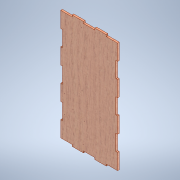
# Autodesk Inventor part: Costados pequeños
Saved by Autodesk Inventor 2020.3 (Build 243373000, 373)
## iProperties
Created: 2020-04-27
Part Number: Costados pequeños
Material: Madera (roble)
Document SubType Name: Modeling
Designer: miosh
Density: 0.76 g/cm^3
Appearance: Roble blanco - Natural brillo medio
Author: miosh
Autodesk Inventor part; units mm, degrees
ref_plane "YZ Plane" through (0, 0, 0) normal (1, 0, 0) x (0, 1, 0)
ref_plane "XZ Plane" through (0, 0, 0) normal (0, 1, 0) x (-1, 0, 0)
ref_plane "XY Plane" through (0, 0, 0) normal (0, 0, 1) x (1, 0, 0)
sketch "Boceto1" plane through (0, 0, 0) normal (0, 0, 1) x (1, 0, 0)
  line L0 (20, 0) -> (20, 3)
  line L1 (20, 3) -> (0, 3)
  line L2 (0, 3) -> (0, 30.71)
  line L3 (0, 30.71) -> (3, 30.71)
  line L4 (3, 30.71) -> (3, 58.43)
  line L5 (3, 58.43) -> (0, 58.43)
  line L6 (0, 58.43) -> (0, 86.14)
  line L7 (0, 86.14) -> (3, 86.14)
  line L8 (3, 86.14) -> (3, 113.86)
  line L9 (3, 113.86) -> (0, 113.86)
  line L10 (0, 113.86) -> (0, 141.57)
  line L11 (0, 141.57) -> (3, 141.57)
  line L12 (3, 141.57) -> (3, 169.29)
  line L13 (3, 169.29) -> (0, 169.29)
  line L14 (0, 169.29) -> (0, 197)
  line L15 (0, 197) -> (20, 197)
  line L16 (20, 197) -> (20, 200)
  line L17 (20, 200) -> (40, 200)
  line L18 (40, 200) -> (40, 197)
  line L19 (40, 197) -> (60, 197)
  line L20 (60, 197) -> (60, 200)
  line L21 (60, 200) -> (80, 200)
  line L22 (80, 200) -> (80, 197)
  line L23 (80, 197) -> (100, 197)
  line L24 (100, 197) -> (100, 169.29)
  line L25 (100, 169.29) -> (97, 169.29)
  line L26 (97, 169.29) -> (97, 141.57)
  line L27 (97, 141.57) -> (100, 141.57)
  line L28 (100, 141.57) -> (100, 113.86)
  line L29 (100, 113.86) -> (97, 113.86)
  line L30 (97, 113.86) -> (97, 86.14)
  line L31 (97, 86.14) -> (100, 86.14)
  line L32 (100, 86.14) -> (100, 58.43)
  line L33 (100, 58.43) -> (97, 58.43)
  line L34 (97, 58.43) -> (97, 30.71)
  line L35 (97, 30.71) -> (100, 30.71)
  line L36 (100, 30.71) -> (100, 3)
  line L37 (100, 3) -> (80, 3)
  line L38 (80, 3) -> (80, 0)
  line L39 (80, 0) -> (60, 0)
  line L40 (60, 0) -> (60, 3)
  line L41 (60, 3) -> (40, 3)
  line L42 (40, 3) -> (40, 0)
  line L43 (40, 0) -> (20, 0)
  point P0 (0, 0)
  dimension "d0" = 3
  dimension "d1" = 27.71
  dimension "d2" = 3
  dimension "d3" = 27.72
  dimension "d4" = 3
  dimension "d5" = 27.71
  dimension "d6" = 3
  dimension "d7" = 27.72
  dimension "d8" = 3
  dimension "d9" = 27.71
  dimension "d10" = 3
  dimension "d11" = 27.72
  dimension "d12" = 3
  dimension "d13" = 27.71
  dimension "d14" = 20
  dimension "d16" = 20
  dimension "d18" = 20
  dimension "d20" = 20
  dimension "d22" = 20
  dimension "d23" = 27.71
  dimension "d24" = 3
  dimension "d25" = 27.72
  dimension "d26" = 3
  dimension "d27" = 27.71
  dimension "d28" = 3
  dimension "d29" = 27.72
  dimension "d30" = 3
  dimension "d31" = 27.71
  dimension "d32" = 3
  dimension "d33" = 27.72
  dimension "d34" = 3
  dimension "d35" = 20
  dimension "d39" = 20
  dimension "d46" = 3
  dimension "d47" = 27.71
  dimension "d50" = 3
  constraints: 88 end point, 26 point on line, 13 perpendicular, 4 vertical, 1 horizontal
  measures "d0" distance of L0.start L0.end
  measures "d1" distance of L1.end L2.end
  measures "d2" distance of L2.end L3.end
  measures "d3" distance of L3.end L4.end
  measures "d4" distance of L4.end L5.end
  measures "d5" distance of L5.end L6.end
  measures "d6" distance of L6.end L7.end
  measures "d7" distance of L7.end L8.end
  measures "d8" distance of L8.end L9.end
  measures "d9" distance of L9.end L10.end
  measures "d10" distance of L10.end L11.end
  measures "d11" distance of L11.end L12.end
  measures "d12" distance of L12.end L13.end
  measures "d13" distance of L13.end L14.end
  measures "d14" distance of L14.end L15.end
  measures "d16" distance of L16.end L17.end
  measures "d18" distance of L18.end L19.end
  measures "d20" distance of L20.end L21.end
  measures "d22" distance of L22.end L23.end
  measures "d23" distance of L23.end L24.end
  measures "d24" distance of L24.end L25.end
  measures "d25" distance of L25.end L26.end
  measures "d26" distance of L26.end L27.end
  measures "d27" distance of L27.end L28.end
  measures "d28" distance of L28.end L29.end
  measures "d29" distance of L29.end L30.end
  measures "d30" distance of L30.end L31.end
  measures "d31" distance of L31.end L32.end
  measures "d32" distance of L32.end L33.end
  measures "d33" distance of L33.end L34.end
  measures "d34" distance of L34.end L35.end
  measures "d35" distance of L36.end L37.end
  measures "d39" distance of L40.end L41.end
  measures "d46" distance of L41.end L42.end
  measures "d47" distance of L35.end L36.end
  measures "d50" distance between parallel lines of L19 L17
extrude "Extrusión1" add sketch "Boceto1" along normal blind 3
